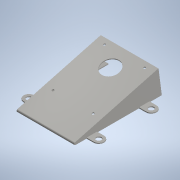
# Autodesk Inventor part: Soporte_LíDAR
Saved by Autodesk Inventor 2022.1 (Build 261234000, 234)
## iProperties
Part Number: Soporte_LíDAR
Material: Genérico
Document SubType Name: Modelado
Designer: seb_0
Appearance: Acero
Author: seb_0
Autodesk Inventor part; units mm, degrees
ref_plane "Plano YZ" through (0, 0, 0) normal (1, 0, 0) x (0, 1, 0)
ref_plane "Plano XZ" through (0, 0, 0) normal (0, 1, 0) x (-1, 0, 0)
ref_plane "Plano XY" through (0, 0, 0) normal (0, 0, 1) x (1, 0, 0)
sketch "Boceto1" plane through (0, 0, 0) normal (1, 0, 0) x (0, 1, 0)
  line L0 (0, -11.3936) -> (0, -110)
  line L1 (0, -110) -> (1, -110)
  line L2 (1, -110) -> (1, -18.9894)
  line L3 (2.9489, -11.0054) -> (28.4701, -106.2518)
  line L4 (28.4701, -106.2518) -> (27.5042, -106.5107)
  line L5 (27.5042, -106.5107) -> (3.9489, -18.6012)
  arc A0 (3.9489, -18.6012) -> (1, -18.9894) centre (2.5, -18.9894) ccw
  arc A1 (2.9489, -11.0054) -> (0, -11.3936) centre (1.5, -11.3936) ccw
  point P0 (0, 0)
  dimension "d0" = 1
  dimension "d1" = 1
  dimension "d2" = 15
  dimension "d3" = 110
  dimension "d4" = 110
  dimension "d5" = 1.5
  constraints: 12 end point, 4 perpendicular, 4 point on circle, 4 tangent, 2 centre point, 2 point on line, 1 equal radius, 1 vertical
  measures "d0" distance of L0.end L1.end
  measures "d1" distance of L3.end L4.end
  measures "d2" angle of L2 L5
  measures "d3" distance of point (0, 0) L0.end
  measures "d4" distance of point (0, 0) L3.end
  measures "d5" radius of A0
extrude "Extrusión1" add sketch "Boceto1" along normal blind 64
sketch "Boceto3" plane through (64, 0, 0) normal (1, 0, 0) x (0, 0, -1)
  line L0 (11.3936, 0) -> (110, 0) projected
  line L1 (110, 0) -> (110, 1) projected
  line L2 (110, 1) -> (18.9894, 1) projected
  arc A0 (18.6012, 3.9489) -> (18.9894, 1) centre (18.9894, 2.5) ccw projected
  line L3 (18.6012, 3.9489) -> (106.5107, 27.5042) projected
  line L4 (106.5107, 27.5042) -> (106.2518, 28.4701) projected
  line L5 (106.2518, 28.4701) -> (11.0054, 2.9489) projected
  arc A1 (11.0054, 2.9489) -> (11.3936, 0) centre (11.3936, 1.5) ccw projected
  line L6 (106.5107, 27.5042) -> (110, 1)
  point P0 (0, 0)
  constraints: 2 end point
extrude "Extrusión2" add sketch "Boceto3" along normal blind 1
sketch "Boceto4" plane through (0, 0, 0) normal (-1, 0, 0) x (0, 0, 1)
  line L0 (-11.3936, 0) -> (-110, 0) projected
  arc A0 (-11.3936, 0) -> (-11.0054, 2.9489) centre (-11.3936, 1.5) ccw projected
  line L1 (-106.2518, 28.4701) -> (-11.0054, 2.9489) projected
  line L2 (-106.5107, 27.5042) -> (-106.2518, 28.4701) projected
  line L3 (-18.6012, 3.9489) -> (-106.5107, 27.5042) projected
  arc A1 (-18.9894, 1) -> (-18.6012, 3.9489) centre (-18.9894, 2.5) ccw projected
  line L4 (-110, 1) -> (-18.9894, 1) projected
  line L5 (-110, 0) -> (-110, 1) projected
  line L6 (-110, 1) -> (-106.5107, 27.5042) projected
  point P0 (0, 0)
extrude "Extrusión3" add sketch "Boceto4" along normal blind 1
sketch "Boceto5" plane through (-1, 2.9489, -11.0054) normal (0, 0.9659258, 0.258819) x (1, 0, 0)
  circle A0 centre (10, 92.6064) radius 1.25
  circle A1 centre (56, 92.6064) radius 1.25
  circle A2 centre (10, 31.6064) radius 1.25
  circle A3 centre (56, 31.6064) radius 1.25
  line L0 (0, 98.6064) -> (66, 98.6064) projected
  line L1 (0, 0) -> (0, 98.6064) projected
  line L2 (10, 92.6064) -> (56, 92.6064)
  line L3 (56, 92.6064) -> (56, 31.6064)
  line L4 (56, 31.6064) -> (10, 31.6064)
  line L5 (10, 31.6064) -> (10, 92.6064)
  circle A4 centre (32, 76.9064) radius 10
  point P0 (1, -11.3936)
  dimension "d12" = 2.5
  dimension "d17" = 46
  dimension "d18" = 10
  dimension "d19" = 61
  dimension "d20" = 6
  dimension "d23" = 20
  dimension "d24" = 21.7
  dimension "d25" = 32
  constraints: 8 end point, 5 centre point, 3 equal radius, 2 horizontal, 2 vertical
  measures "d12" diameter of A0
  measures "d17" distance of L2.start L2.end
  measures "d18" distance between parallel lines of L1 L5
  measures "d19" distance of L2.end L3.end
  measures "d20" distance between parallel lines of L2 L0
  measures "d23" diameter of A4
  measures "d24" distance from line of L0 A4.centre
  measures "d25" distance from line of L1 A4.centre
extrude "Extrusión4" cut sketch "Boceto5" against normal blind 1 contours L2 L5 A0 | A0 L5 L2 | L2 L3 A1 | A1 L3 L2 | L5 L4 A2 | A2 L4 L5 | L3 L4 A3 | A3 L4 L3 | A4
sketch "Boceto6" plane through (65, 0, -110) normal (0, -1, 0) x (1, 0, 0)
  line L0 (0, 98.6064) -> (0, 0) projected
  line L1 (-66, 0) -> (-66, 98.6064) projected
  line L2 (-5, 98.6064) -> (-5, 0)
  line L3 (-61, 0) -> (-61, 98.6064)
  line L4 (-66, 100.1064) -> (0, 100.1064) projected
  line L5 (-66, 90.1064) -> (0, 90.1064)
  line L6 (-66, 0) -> (0, 0) projected
  line L7 (0, 98.6064) -> (0, 0) projected
  line L8 (0, 98.6064) -> (-66, 98.6064) projected
  line L9 (-66, 0) -> (-66, 98.6064) projected
  point P0 (-5, 90.1064)
  point P1 (-61, 90.1064)
  dimension "d29" = 5
  dimension "d30" = 5
  dimension "d31" = 10
  constraints: 6 end point, 3 parallel
  measures "d29" distance between parallel lines of L0 L2
  measures "d30" distance between parallel lines of L1 L3
  measures "d31" distance between parallel lines of L4 L5
extrude "Extrusión5" cut sketch "Boceto6" against normal blind 1 contours L2 L6 L3 L5
sketch "Boceto7" plane through (65, 0, -110) normal (0, -1, 0) x (1, 0, 0)
  circle A0 centre (8, 80) radius 3
  circle A1 centre (8, 20) radius 3
  circle A2 centre (-72, 80) radius 3
  circle A3 centre (-72, 20) radius 3
  line L0 (-72, 80) -> (8, 80)
  line L1 (8, 80) -> (8, 20)
  line L2 (8, 20) -> (-72, 20)
  line L3 (-72, 20) -> (-72, 80)
  line L4 (-5, 0) -> (0, 0) projected
  line L5 (0, 98.6064) -> (0, 0) projected
  circle A4 centre (8, 80) radius 6
  circle A5 centre (8, 20) radius 6
  circle A6 centre (-72, 20) radius 6
  circle A7 centre (-72, 80) radius 6
  line L6 (8, 86) -> (0, 86)
  line L7 (8, 74) -> (0, 74)
  line L8 (8, 26) -> (0, 26)
  line L9 (8, 14) -> (0, 14)
  line L10 (-72, 86) -> (-66, 86)
  line L11 (-66, 98.9946) -> (-66, 3.7482) projected
  line L12 (-72, 74) -> (-66, 74)
  line L13 (-72, 14) -> (-66, 14)
  line L14 (-72, 26) -> (-66, 26)
  point P0 (-65, 110)
  dimension "d32" = 6
  dimension "d36" = 80
  dimension "d37" = 60
  dimension "d38" = 20
  dimension "d39" = 8
  dimension "d40" = 3
  dimension "d41" = 3
  dimension "d42" = 3
  dimension "d43" = 3
  constraints: 24 end point, 18 point on line, 8 centre point, 8 point on circle, 5 parallel, 4 tangent, 3 equal radius, 2 perpendicular, 1 horizontal
  measures "d32" diameter of A0
  measures "d36" distance of L0.start L0.end
  measures "d37" distance of L0.end L1.end
  measures "d38" distance between parallel lines of L4 L2
  measures "d39" distance between parallel lines of L5 L1
  measures "d40" radial gap between concentric circles of A0 A4
  measures "d41" radial gap between concentric circles of A1 A5
  measures "d42" radial gap between concentric circles of A3 A6
  measures "d43" radial gap between concentric circles of A2 A7
extrude "Extrusión6" add sketch "Boceto7" against normal blind 1 contours A0 L0 A4 L1 | A0 L1 A4 L0 | A4 L7 L5 L0 | L0 L5 L6 A4 | A5 L2 A1 L1 | L1 A1 L2 A5 | A5 L2 L5 L8 | A7 L3 A2 L0 | L0 A2 L3 A7 | L11 L12 A7 | A7 L10 L11 | A5 L9 L5 L2 | A6 L2 A3 L3 | L14 L11 A6 | L3 A3 L2 A6 | L11 L13 A6
